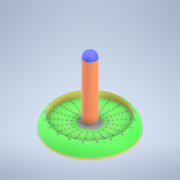
# Autodesk Inventor part: Bottum
Saved by Autodesk Inventor 2021 (Build 250183000, 183)
## iProperties
Created: 2021-07-30
Part Number: Bottum
Material: PVC, Unplasticized
Document SubType Name: Modeling
Designer: Shammy Haider
Density: 1.29 g/cm^3
Appearance: Smooth - White
Author: Shammy Haider
Autodesk Inventor part; units mm, degrees
ref_plane "YZ Plane" through (0, 0, 0) normal (1, 0, 0) x (0, 1, 0)
ref_plane "XZ Plane" through (0, 0, 0) normal (0, 1, 0) x (-1, 0, 0)
ref_plane "XY Plane" through (0, 0, 0) normal (0, 0, 1) x (1, 0, 0)
sketch "Sketch1" plane through (0, 0, 0) normal (0, 1, 0) x (-1, 0, 0)
  circle A0 centre (0, 0) radius 6
  dimension "d0" = 12
  constraints: 1 centre point, 1 coincident
  measures "d0" diameter of A0
extrude "Extrusion1" add sketch "Sketch1" along normal blind 2
shell "Shell1" thickness 1 removed faces 1 at (0.7092, 2, 1.4219)
fillet "Fillet1" radius 2 1 edges at (6, 2, 0)
sketch "Sketch2" plane through (0, 1, 0) normal (0, 1, 0) x (1, 0, 0)
  circle A0 centre (0, 0) radius 1
  dimension "d5" = 2
  constraints: 1 centre point, 1 coincident
  measures "d5" diameter of A0
extrude "Extrusion2" add sketch "Sketch2" along normal blind 10
fillet "Fillet2" radius 1 1 edges at (-1, 11, 0)
fillet "Fillet3" radius 0.5 1 edges at (-1, 1, 0)
sketch "Sketch3" plane through (0, 0, 0) normal (0, -1, 0) x (1, 0, 0)
  circle A0 centre (2.1, 0) radius 0.1
  point P0 (0, 0)
  dimension "d10" = 0.2
  dimension "d11" = 2.1
  constraints: 1 centre point
  measures "d10" diameter of A0
  measures "d11" distance of point (0, 0) A0.centre
extrude "Extrusion3" cut sketch "Sketch3" against normal blind 10
pattern_circular "Circular Pattern1" count 20 over 360 about axis through (0, 0, 0) along (0, -1, 0) of "Extrusion3"
sketch "Sketch4" plane through (0, 0, 0) normal (0, -1, 0) x (1, 0, 0)
  circle A0 centre (0, 2.6463) radius 0.1
  circle A1 centre (0, 0) radius 1 projected
  line L0 (0, 0) -> (0, 5.3051)
  circle A2 centre (0, 3.1463) radius 0.1
  circle A3 centre (0, 3.6463) radius 0.1
  circle A4 centre (0, 4.1463) radius 0.1
  circle A5 centre (0, 4.6463) radius 0.1
  circle A6 centre (0, 5.1463) radius 0.1
  dimension "d17" = 0.2
  dimension "d20" = 0.5
  constraints: 6 centre point, 2 end point, 2 vertical, 10 other
  measures "d17" diameter of A0
  measures "d20" distance of A0.centre A2.centre
extrude "Extrusion4" cut sketch "Sketch4" against normal blind 10 contours A0 L0 | L0 A0 | A2 L0 | L0 A2 | A3 L0 | L0 A3 | A4 L0 | L0 A4 | A5 L0 | L0 A5 | A6 L0 | L0 A6
pattern_circular "Circular Pattern2" count 20 over 360 about axis through (0, 0, 0) along (0, 1, 0) of "Extrusion4"
body "Solid1"
